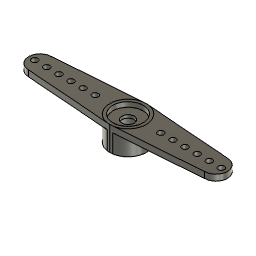
Servo_Motor_Extention (Autodesk Fusion 360 design; units mm, degrees)
Autodesk Fusion 360 part; units mm, degrees
sketch "Sketch1" plane through (0, 0, 0) normal (0, 0, 1) x (1, 0, 0)
  arc A0 (0, 3) -> (0, -3) centre (0, 0) ccw
  line L0 (0, 0) -> (0, 3) construction
  line L1 (0, 0) -> (0, -3) construction
  line L2 (0, 0) -> (23, 0) construction
  arc A1 (14.5, -1.8997) -> (14.5, 1.8997) centre (14.5, 0) ccw
  line L3 (14.5, 0) -> (14.5, -1.8997) construction
  line L4 (14.5, 0) -> (14.5, 1.8997) construction
  line L5 (0, -3) -> (14.5, -1.8997)
  line L6 (14.5, 1.8997) -> (0, 3)
  dimension "d48" = 180
  dimension "d49" = 180
  dimension "d50" = 14.5
  constraint coincident A0.centre L0.start
  constraint perpendicular L0 L2
  constraint coincident L2 A1.centre
  measures "d48" angle of L0 L1
  measures "d49" angle of L3 L4
  measures "d50" distance of A0.centre A1.centre
extrude "Extrude1" add sketch "Sketch1" along normal blind 1 makes body 1
sketch "Sketch2" plane through (0, 0, 1) normal (0, 0, 1) x (-1, 0, 0)
  line L0 (-14.5, -1.8997) -> (0, -3)
  arc A0 (0, -3) -> (0, 3) centre (0, 0) ccw
  line L1 (0, 3) -> (-14.5, 1.8997)
  arc A1 (-14.5, 1.8997) -> (-14.5, -1.8997) centre (-14.5, 0) ccw
  circle A2 centre (0, 0) radius 2.5
  dimension "d53" = 5
  constraint coincident A0.centre A2.centre
  measures "d53" diameter of A2
extrude "Extrude2" cut sketch "Sketch2" against normal blind 0.8 contours A2 bodies 1
sketch "Sketch3" plane through (0, 0, 0) normal (0, 0, -1) x (1, 0, 0)
  line L0 (0, -3) -> (14.5, -1.8997)
  arc A0 (14.5, -1.8997) -> (14.5, 1.8997) centre (14.5, 0) ccw
  line L1 (14.5, 1.8997) -> (0, 3)
  arc A1 (0, 3) -> (0, -3) centre (0, 0) ccw
  circle A2 centre (0, 0) radius 3
  dimension "d56" = 6
  constraint coincident A1.centre A2.centre
  measures "d56" diameter of A2
extrude "Extrude3" add sketch "Sketch3" along normal blind 3 contours L0 L1 A1 A2 bodies 1
sketch "Sketch4" plane through (0, 0, -3) normal (0, 0, -1) x (1, 0, 0)
  arc A0 (0.4527, -2.9656) -> (0.4527, 2.9656) centre (0, 0) ccw
  line L0 (0.4527, 2.9656) -> (0, 3)
  arc A1 (0, 3) -> (0, -3) centre (0, 0) ccw
  line L1 (0, -3) -> (0.4527, -2.9656)
  circle A2 centre (0, 0) radius 2.3
  dimension "d59" = 4.6
  constraint coincident A0.centre A1.centre
  measures "d59" diameter of A2
extrude "Extrude4" cut sketch "Sketch4" against normal blind 2.7 contours A2 bodies 1
sketch "Sketch5" plane through (0, 0, 0.2) normal (0, 0, 1) x (-1, 0, 0)
  circle A0 centre (0, 0) radius 2.5
  circle A1 centre (0, 0) radius 1
  dimension "d62" = 2
  constraint coincident A0.centre A1.centre
  measures "d62" diameter of A1
extrude "Extrude5" cut sketch "Sketch5" against normal up to surface (0.5 mm away) contours A1 bodies 1
sketch "Sketch6" plane through (0, 0, 1) normal (0, 0, 1) x (-1, 0, 0)
  circle A0 centre (0, 0) radius 2.5
  line L0 (-14.5, -1.8997) -> (0, -3)
  arc A1 (0, -3) -> (0, 3) centre (0, 0) ccw
  line L1 (0, 3) -> (-14.5, 1.8997)
  arc A2 (-14.5, 1.8997) -> (-14.5, -1.8997) centre (-14.5, 0) ccw
  line L2 (0, 0) -> (-18.6783, 0) construction
  circle A3 centre (-15.4, 0) radius 0.5
  circle A4 centre (-13.4, 0) radius 0.5
  circle A5 centre (-11.4, 0) radius 0.5
  circle A6 centre (-9.4, 0) radius 0.5
  circle A7 centre (-7.4, 0) radius 0.5
  circle A8 centre (-5.4, 0) radius 0.5
  dimension "d65" = 1
  dimension "d66" = 15.4
  dimension "d67" = 1
  dimension "d68" = 2
  dimension "d69" = 1
  dimension "d70" = 2
  dimension "d71" = 1
  dimension "d72" = 2
  dimension "d73" = 1
  dimension "d74" = 2
  dimension "d75" = 1
  dimension "d76" = 2
  constraint coincident A0.centre A1.centre
  constraint horizontal L2
  constraint coincident L2 A3.centre
  constraint coincident L2 A4.centre
  constraint coincident L2 A5.centre
  constraint coincident L2 A6.centre
  constraint coincident L2 A7.centre
  constraint coincident L2 A8.centre
  measures "d65" diameter of A3
  measures "d66" distance of A0.centre A3.centre
  measures "d67" diameter of A4
  measures "d68" distance of A3.centre A4.centre
  measures "d69" diameter of A5
  measures "d70" distance of A4.centre A5.centre
  measures "d71" diameter of A6
  measures "d72" distance of A5.centre A6.centre
  measures "d73" diameter of A7
  measures "d74" distance of A6.centre A7.centre
  measures "d75" diameter of A8
  measures "d76" distance of A7.centre A8.centre
extrude "Extrude6" cut sketch "Sketch6" against normal up to surface (1 mm away) contours A3 | A4 | A5 | A6 | A7 | A8 bodies 1
mirror "Mirror1" about plane through (0, 0, 0) normal (1, 0, 0) of "Extrude1", "Extrude2", "Extrude3", "Extrude4", "Extrude5", "Extrude6" makes body 2
